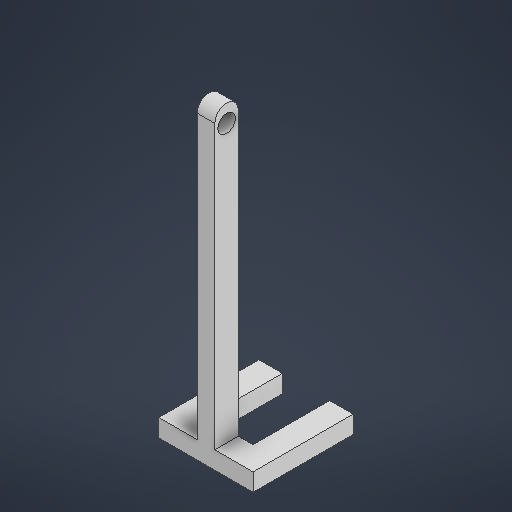
# Autodesk Inventor part: Soporte_Seguro_Tapa
Saved by Autodesk Inventor 2026 (Build 300175000, 175)
## iProperties
Created: 2025-07-02
Part Number: Soporte_Seguro_Tapa
Material: Genérico
Document SubType Name: Modeling
Designer: oscar
Density: 1 g/cm^3
Appearance: Valor por defecto
Author: oscar
Autodesk Inventor part; units mm, degrees
ref_plane "YZ Plane" through (0, 0, 0) normal (1, 0, 0) x (0, 1, 0)
ref_plane "XZ Plane" through (0, 0, 0) normal (0, 1, 0) x (-1, 0, 0)
ref_plane "XY Plane" through (0, 0, 0) normal (0, 0, 1) x (1, 0, 0)
sketch "Boceto1" plane through (0, 0, 0) normal (0, 1, 0) x (-1, 0, 0)
  line L0 (-8, 5.1855) -> (-8, -11.8145)
  line L1 (-8, -11.8145) -> (-4, -11.8145)
  line L2 (-4, -11.8145) -> (-4, 1.1855)
  line L3 (-4, 1.1855) -> (4, 1.1855)
  line L4 (4, 1.1855) -> (4, -11.8145)
  line L5 (4, -11.8145) -> (8, -11.8145)
  line L6 (8, -11.8145) -> (8, 5.1855)
  line L7 (8, 5.1855) -> (-8, 5.1855)
  point P0 (3.454, 5.1855)
  dimension "d1" = 8
  dimension "d2" = 13
  dimension "d3" = 13
  dimension "d4" = 4
  dimension "d5" = 4
  dimension "d6" = 4
  constraints: 16 end point, 6 perpendicular, 1 horizontal
  measures "d1" distance of L2.end L3.end
  measures "d2" distance of L3.end L4.end
  measures "d3" distance of L1.end L2.end
  measures "d4" distance of L4.end L5.end
  measures "d5" distance of L0.end L1.end
  measures "d6" distance from line of L3 point (3.454, 5.185)
extrude "Extrusión1" add sketch "Boceto1" along normal blind 3
sketch "Boceto2" plane through (0, 3, 0) normal (0, 1, 0) x (1, 0, 0)
  line L0 (-8, -5.1855) -> (8, -5.1855) projected
  line L1 (4, -1.1855) -> (-4, -1.1855) projected
  line L2 (-1.5, -5.1855) -> (1.5, -5.1855)
  line L3 (1.5, -5.1855) -> (1.5, -1.1855)
  line L4 (1.5, -1.1855) -> (-1.5, -1.1855)
  line L5 (-1.5, -1.1855) -> (-1.5, -5.1855)
  line L6 (-8, 11.8145) -> (-8, -5.1855) projected
  point P0 (0, 0)
  point P1 (-1.5, -3.1855)
  point P2 (0, -3.2062)
  point P3 (-1.5, -1.1855)
  dimension "d10" = 3
  dimension "d13" = 1.5
  dimension "d14" = 6.5
  constraints: 8 end point, 2 parallel, 2 point on line, 1 horizontal, 1 midpoint, 1 perpendicular
  measures "d10" distance of L4.end L3.end
  measures "d13" horizontal distance of point (-1.5, -3.185) point (0, -3.206)
  measures "d14" distance between parallel lines of L6 L5
extrude "Extrusión2" add sketch "Boceto2" along normal blind 50
fillet "Empalme1" radius 2 2 edges at (0, 53, 1.1855) (0, 53, 5.1855)
sketch "Boceto3" plane through (-1.5, 3, 1.1855) normal (-1, 0, 0) x (0, 0, 1)
  circle A0 centre (2, 47) radius 1.5
  line L0 (0, 0) -> (0, 48) projected
  arc A1 (4, 48) -> (0, 48) centre (2, 48) ccw projected
  point P0 (-1.1855, -3)
  dimension "d18" = 3
  dimension "d19" = 2
  dimension "d20" = 1
  constraints: 1 centre point
  measures "d18" diameter of A0
  measures "d19" distance from line of L0 A0.centre
  measures "d20" distance of A1.centre A0.centre
extrude "Extrusión3" cut sketch "Boceto3" against normal blind 25
sketch "Boceto5" plane through (-1.5, 3, 1.1855) normal (-1, 0, 0) x (0, 0, 1)
  line L0 (4, 0) -> (4, 48) projected
  line L1 (0, 0) -> (0, 48) projected
  line L2 (0, 41.0837) -> (0, 5.7835)
  line L3 (4, 5.7835) -> (4, 41.0837)
  spline S0 degree 2 poles (1.1837, 10.435) (1.2834, 10.5201) (1.5751, 10.6149) (1.7623, 10.6149) knots 0 0 0 1 2 2 2
  spline S1 degree 2 poles (1.7623, 10.6149) (1.9446, 10.6149) (2.24, 10.5225) (2.3397, 10.435) knots 0 0 0 1 2 2 2
  spline S2 degree 2 poles (2.3397, 10.435) (2.4442, 10.3426) (2.5439, 10.0983) (2.5439, 9.9512) knots 0 0 0 1 2 2 2
  spline S3 degree 2 poles (2.5439, 9.9512) (2.5439, 9.7992) (2.4406, 9.5561) (2.3397, 9.4674) knots 0 0 0 1 2 2 2
  spline S4 degree 2 poles (2.3397, 9.4674) (2.24, 9.3811) (1.9471, 9.2887) (1.7623, 9.2887) knots 0 0 0 1 2 2 2
  spline S5 degree 2 poles (1.7623, 9.2887) (1.5739, 9.2887) (1.287, 9.3823) (1.1837, 9.4686) knots 0 0 0 1 2 2 2
  spline S6 degree 2 poles (1.1837, 9.4686) (1.084, 9.5561) (0.9807, 9.8004) (0.9807, 9.9512) knots 0 0 0 1 2 2 2
  spline S7 degree 2 poles (0.9807, 9.9512) (0.9807, 10.1043) (1.0877, 10.3499) (1.1837, 10.435) knots 0 0 0 1 2 2 2
  spline S8 degree 2 poles (1.7623, 10.407) (1.614, 10.407) (1.3843, 10.3426) (1.3089, 10.2842) knots 0 0 0 1 2 2 2
  spline S9 degree 2 poles (1.3089, 10.2842) (1.2311, 10.2247) (1.1533, 10.0569) (1.1533, 9.9524) knots 0 0 0 1 2 2 2
  spline S10 degree 2 poles (1.1533, 9.9524) (1.1533, 9.8442) (1.2287, 9.6813) (1.3089, 9.6193) knots 0 0 0 1 2 2 2
  spline S11 degree 2 poles (1.3089, 9.6193) (1.3855, 9.5598) (1.6164, 9.4966) (1.7623, 9.4966) knots 0 0 0 1 2 2 2
  spline S12 degree 2 poles (1.7623, 9.4966) (2.0577, 9.4966) (2.3713, 9.7445) (2.3713, 9.9524) knots 0 0 0 1 2 2 2
  spline S13 degree 2 poles (2.3713, 9.9524) (2.3713, 10.1603) (2.0577, 10.407) (1.7623, 10.407) knots 0 0 0 1 2 2 2
  spline S14 degree 2 poles (2.539, 11.2518) (2.539, 11.0889) (2.471, 10.8604) (2.4223, 10.7595) knots 0 0 0 1 2 2 2
  line L4 (2.4223, 10.7595) -> (2.1719, 10.7595)
  line L5 (2.1719, 10.7595) -> (2.1719, 10.7741)
  spline S15 degree 2 poles (2.1719, 10.7741) (2.2643, 10.8726) (2.3664, 11.1218) (2.3664, 11.2372) knots 0 0 0 1 2 2 2
  spline S16 degree 2 poles (2.3664, 11.2372) (2.3664, 11.4026) (2.2291, 11.5715) (2.116, 11.5715) knots 0 0 0 1 2 2 2
  spline S17 degree 2 poles (2.116, 11.5715) (2.0261, 11.5715) (1.9142, 11.4828) (1.8863, 11.3867) knots 0 0 0 1 2 2 2
  spline S18 degree 2 poles (1.8863, 11.3867) (1.8668, 11.3175) (1.8401, 11.202) (1.8182, 11.1157) knots 0 0 0 1 2 2 2
  spline S19 degree 2 poles (1.8182, 11.1157) (1.7975, 11.0379) (1.7355, 10.9151) (1.6857, 10.8677) knots 0 0 0 1 2 2 2
  spline S20 degree 2 poles (1.6857, 10.8677) (1.6359, 10.8215) (1.5022, 10.7705) (1.4146, 10.7705) knots 0 0 0 1 2 2 2
  spline S21 degree 2 poles (1.4146, 10.7705) (1.2323, 10.7705) (0.9855, 11.0549) (0.9855, 11.2749) knots 0 0 0 1 2 2 2
  spline S22 degree 2 poles (0.9855, 11.2749) (0.9855, 11.4013) (1.0354, 11.625) (1.0828, 11.721) knots 0 0 0 1 2 2 2
  line L6 (1.0828, 11.721) -> (1.321, 11.721)
  line L7 (1.321, 11.721) -> (1.321, 11.7064)
  spline S23 degree 2 poles (1.321, 11.7064) (1.2554, 11.6347) (1.1582, 11.4111) (1.1582, 11.2883) knots 0 0 0 1 2 2 2
  spline S24 degree 2 poles (1.1582, 11.2883) (1.1582, 11.1497) (1.2882, 10.9783) (1.394, 10.9783) knots 0 0 0 1 2 2 2
  spline S25 degree 2 poles (1.394, 10.9783) (1.4888, 10.9783) (1.6018, 11.0792) (1.6274, 11.174) knots 0 0 0 1 2 2 2
  spline S26 degree 2 poles (1.6274, 11.174) (1.6444, 11.2372) (1.6881, 11.4208) (1.7064, 11.4816) knots 0 0 0 1 2 2 2
  spline S27 degree 2 poles (1.7064, 11.4816) (1.7538, 11.6359) (1.9446, 11.7794) (2.0844, 11.7794) knots 0 0 0 1 2 2 2
  spline S28 degree 2 poles (2.0844, 11.7794) (2.1731, 11.7794) (2.3433, 11.7077) (2.4029, 11.6432) knots 0 0 0 1 2 2 2
  spline S29 degree 2 poles (2.4029, 11.6432) (2.4685, 11.5715) (2.539, 11.3892) (2.539, 11.2518) knots 0 0 0 1 2 2 2
  spline S30 degree 2 poles (2.539, 12.5683) (2.539, 12.4224) (2.4406, 12.1756) (2.3421, 12.0857) knots 0 0 0 1 2 2 2
  spline S31 degree 2 poles (2.3421, 12.0857) (2.2449, 11.9957) (1.9531, 11.8973) (1.7635, 11.8973) knots 0 0 0 1 2 2 2
  spline S32 degree 2 poles (1.7635, 11.8973) (1.5751, 11.8973) (1.2955, 11.9933) (1.1922, 12.0845) knots 0 0 0 1 2 2 2
  spline S33 degree 2 poles (1.1922, 12.0845) (1.0913, 12.1744) (0.9855, 12.42) (0.9855, 12.5719) knots 0 0 0 1 2 2 2
  spline S34 degree 2 poles (0.9855, 12.5719) (0.9855, 12.6473) (1.0074, 12.7798) (1.0244, 12.8357) knots 0 0 0 1 2 2 2
  spline S35 degree 2 poles (1.0244, 12.8357) (1.0402, 12.8843) (1.0852, 12.9852) (1.112, 13.035) knots 0 0 0 1 2 2 2
  line L8 (1.112, 13.035) -> (1.3526, 13.035)
  line L9 (1.3526, 13.035) -> (1.3526, 13.0192)
  spline S36 degree 2 poles (1.3526, 13.0192) (1.3283, 12.9925) (1.2603, 12.9098) (1.2274, 12.8503) knots 0 0 0 1 2 2 2
  spline S37 degree 2 poles (1.2274, 12.8503) (1.1958, 12.7932) (1.1557, 12.6582) (1.1557, 12.5707) knots 0 0 0 1 2 2 2
  spline S38 degree 2 poles (1.1557, 12.5707) (1.1557, 12.4747) (1.2347, 12.3033) (1.3101, 12.2389) knots 0 0 0 1 2 2 2
  spline S39 degree 2 poles (1.3101, 12.2389) (1.3867, 12.1756) (1.6189, 12.1051) (1.7635, 12.1051) knots 0 0 0 1 2 2 2
  spline S40 degree 2 poles (1.7635, 12.1051) (1.9179, 12.1051) (2.1403, 12.1793) (2.2169, 12.2437) knots 0 0 0 1 2 2 2
  spline S41 degree 2 poles (2.2169, 12.2437) (2.2911, 12.3069) (2.3664, 12.4759) (2.3664, 12.5707) knots 0 0 0 1 2 2 2
  spline S42 degree 2 poles (2.3664, 12.5707) (2.3664, 12.657) (2.3239, 12.8041) (2.2923, 12.8612) knots 0 0 0 1 2 2 2
  spline S43 degree 2 poles (2.2923, 12.8612) (2.2607, 12.9159) (2.195, 12.9974) (2.1719, 13.0205) knots 0 0 0 1 2 2 2
  line L10 (2.1719, 13.0205) -> (2.1719, 13.035)
  line L11 (2.1719, 13.035) -> (2.4102, 13.035)
  spline S44 degree 2 poles (2.4102, 13.035) (2.4333, 12.9852) (2.4758, 12.8977) (2.4953, 12.8357) knots 0 0 0 1 2 2 2
  spline S45 degree 2 poles (2.4953, 12.8357) (2.5172, 12.7701) (2.539, 12.6582) (2.539, 12.5683) knots 0 0 0 1 2 2 2
  line L12 (2.5123, 13.0594) -> (1.0123, 13.565)
  line L13 (1.0123, 13.565) -> (1.0123, 13.8106)
  line L14 (1.0123, 13.8106) -> (2.5123, 14.3162)
  line L15 (2.5123, 14.3162) -> (2.5123, 14.106)
  line L16 (2.5123, 14.106) -> (2.0929, 13.9698)
  line L17 (2.0929, 13.9698) -> (2.0929, 13.3973)
  line L18 (2.0929, 13.3973) -> (2.5123, 13.2611)
  line L19 (2.5123, 13.2611) -> (2.5123, 13.0594)
  line L20 (1.9227, 13.9151) -> (1.2165, 13.6829)
  line L21 (1.2165, 13.6829) -> (1.9227, 13.452)
  line L22 (1.9227, 13.452) -> (1.9227, 13.9151)
  line L23 (2.5123, 15.6388) -> (2.5123, 15.3799)
  line L24 (2.5123, 15.3799) -> (1.9155, 14.9058)
  line L25 (1.9155, 14.9058) -> (1.9155, 14.6773)
  line L26 (1.9155, 14.6773) -> (2.5123, 14.6773)
  line L27 (2.5123, 14.6773) -> (2.5123, 14.4779)
  line L28 (2.5123, 14.4779) -> (1.0123, 14.4779)
  line L29 (1.0123, 14.4779) -> (1.0123, 14.8645)
  spline S46 degree 2 poles (1.0123, 14.8645) (1.0123, 14.9933) (1.0402, 15.1671) (1.0913, 15.2462) knots 0 0 0 1 2 2 2
  spline S47 degree 2 poles (1.0913, 15.2462) (1.1424, 15.3252) (1.3016, 15.4163) (1.4195, 15.4163) knots 0 0 0 1 2 2 2
  spline S48 degree 2 poles (1.4195, 15.4163) (1.5836, 15.4163) (1.8061, 15.2486) (1.8595, 15.1051) knots 0 0 0 1 2 2 2
  line L30 (1.8595, 15.1051) -> (2.5123, 15.6388)
  spline S49 degree 2 poles (1.4353, 15.2085) (1.3697, 15.2085) (1.2688, 15.1623) (1.236, 15.1137) knots 0 0 0 1 2 2 2
  spline S50 degree 2 poles (1.236, 15.1137) (1.208, 15.0711) (1.1849, 14.9581) (1.1849, 14.8754) knots 0 0 0 1 2 2 2
  line L31 (1.1849, 14.8754) -> (1.1849, 14.6773)
  line L32 (1.1849, 14.6773) -> (1.7489, 14.6773)
  line L33 (1.7489, 14.6773) -> (1.7489, 14.8523)
  spline S51 degree 2 poles (1.7489, 14.8523) (1.7489, 14.9386) (1.7185, 15.076) (1.6711, 15.1234) knots 0 0 0 1 2 2 2
  spline S52 degree 2 poles (1.6711, 15.1234) (1.6298, 15.1671) (1.5131, 15.2085) (1.4353, 15.2085) knots 0 0 0 1 2 2 2
  line L34 (2.9073, 16.7279) -> (2.9073, 16.5602)
  line L35 (2.9073, 16.5602) -> (0.9454, 16.5602)
  line L36 (0.9454, 16.5602) -> (0.9454, 16.7279)
  line L37 (0.9454, 16.7279) -> (2.9073, 16.7279)
  line L38 (2.5123, 18.358) -> (2.5123, 17.7769)
  line L39 (2.5123, 17.7769) -> (2.3591, 17.7769)
  line L40 (2.3591, 17.7769) -> (2.3591, 17.9678)
  line L41 (2.3591, 17.9678) -> (1.1655, 17.9678)
  line L42 (1.1655, 17.9678) -> (1.1655, 17.7769)
  line L43 (1.1655, 17.7769) -> (1.0123, 17.7769)
  line L44 (1.0123, 17.7769) -> (1.0123, 18.358)
  line L45 (1.0123, 18.358) -> (1.1655, 18.358)
  line L46 (1.1655, 18.358) -> (1.1655, 18.1671)
  line L47 (1.1655, 18.1671) -> (2.3591, 18.1671)
  line L48 (2.3591, 18.1671) -> (2.3591, 18.358)
  line L49 (2.3591, 18.358) -> (2.5123, 18.358)
  line L50 (2.5123, 19.7656) -> (2.5123, 19.5067)
  line L51 (2.5123, 19.5067) -> (1.9155, 19.0326)
  line L52 (1.9155, 19.0326) -> (1.9155, 18.8041)
  line L53 (1.9155, 18.8041) -> (2.5123, 18.8041)
  line L54 (2.5123, 18.8041) -> (2.5123, 18.6047)
  line L55 (2.5123, 18.6047) -> (1.0123, 18.6047)
  line L56 (1.0123, 18.6047) -> (1.0123, 18.9913)
  spline S53 degree 2 poles (1.0123, 18.9913) (1.0123, 19.1201) (1.0402, 19.294) (1.0913, 19.373) knots 0 0 0 1 2 2 2
  spline S54 degree 2 poles (1.0913, 19.373) (1.1424, 19.452) (1.3016, 19.5432) (1.4195, 19.5432) knots 0 0 0 1 2 2 2
  spline S55 degree 2 poles (1.4195, 19.5432) (1.5836, 19.5432) (1.8061, 19.3754) (1.8595, 19.232) knots 0 0 0 1 2 2 2
  line L57 (1.8595, 19.232) -> (2.5123, 19.7656)
  spline S56 degree 2 poles (1.4353, 19.3353) (1.3697, 19.3353) (1.2688, 19.2891) (1.236, 19.2405) knots 0 0 0 1 2 2 2
  spline S57 degree 2 poles (1.236, 19.2405) (1.208, 19.1979) (1.1849, 19.0849) (1.1849, 19.0022) knots 0 0 0 1 2 2 2
  line L58 (1.1849, 19.0022) -> (1.1849, 18.8041)
  line L59 (1.1849, 18.8041) -> (1.7489, 18.8041)
  line L60 (1.7489, 18.8041) -> (1.7489, 18.9791)
  spline S58 degree 2 poles (1.7489, 18.9791) (1.7489, 19.0654) (1.7185, 19.2028) (1.6711, 19.2502) knots 0 0 0 1 2 2 2
  spline S59 degree 2 poles (1.6711, 19.2502) (1.6298, 19.294) (1.5131, 19.3353) (1.4353, 19.3353) knots 0 0 0 1 2 2 2
  line L61 (2.5123, 21.1708) -> (2.5123, 20.9714)
  line L62 (2.5123, 20.9714) -> (1.2202, 20.9714)
  line L63 (1.2202, 20.9714) -> (2.099, 20.58)
  line L64 (2.099, 20.58) -> (2.099, 20.4585)
  line L65 (2.099, 20.4585) -> (1.2202, 20.0707)
  line L66 (1.2202, 20.0707) -> (2.5123, 20.0707)
  line L67 (2.5123, 20.0707) -> (2.5123, 19.8847)
  line L68 (2.5123, 19.8847) -> (1.0123, 19.8847)
  line L69 (1.0123, 19.8847) -> (1.0123, 20.157)
  line L70 (1.0123, 20.157) -> (1.8474, 20.5314)
  line L71 (1.8474, 20.5314) -> (1.0123, 20.8936)
  line L72 (1.0123, 20.8936) -> (1.0123, 21.1708)
  line L73 (1.0123, 21.1708) -> (2.5123, 21.1708)
  line L74 (2.5123, 21.313) -> (1.0123, 21.8187)
  line L75 (1.0123, 21.8187) -> (1.0123, 22.0642)
  line L76 (1.0123, 22.0642) -> (2.5123, 22.5699)
  line L77 (2.5123, 22.5699) -> (2.5123, 22.3596)
  line L78 (2.5123, 22.3596) -> (2.0929, 22.2235)
  line L79 (2.0929, 22.2235) -> (2.0929, 21.6509)
  line L80 (2.0929, 21.6509) -> (2.5123, 21.5148)
  line L81 (2.5123, 21.5148) -> (2.5123, 21.313)
  line L82 (1.9227, 22.1688) -> (1.2165, 21.9366)
  line L83 (1.2165, 21.9366) -> (1.9227, 21.7056)
  line L84 (1.9227, 21.7056) -> (1.9227, 22.1688)
  line L85 (2.9073, 23.7016) -> (2.9073, 23.5338)
  line L86 (2.9073, 23.5338) -> (0.9454, 23.5338)
  line L87 (0.9454, 23.5338) -> (0.9454, 23.7016)
  line L88 (0.9454, 23.7016) -> (2.9073, 23.7016)
  spline S60 degree 2 poles (2.539, 25.3949) (2.539, 25.249) (2.4406, 25.0022) (2.3421, 24.9123) knots 0 0 0 1 2 2 2
  spline S61 degree 2 poles (2.3421, 24.9123) (2.2449, 24.8223) (1.9531, 24.7239) (1.7635, 24.7239) knots 0 0 0 1 2 2 2
  spline S62 degree 2 poles (1.7635, 24.7239) (1.5751, 24.7239) (1.2955, 24.8199) (1.1922, 24.9111) knots 0 0 0 1 2 2 2
  spline S63 degree 2 poles (1.1922, 24.9111) (1.0913, 25.001) (0.9855, 25.2466) (0.9855, 25.3985) knots 0 0 0 1 2 2 2
  spline S64 degree 2 poles (0.9855, 25.3985) (0.9855, 25.4739) (1.0074, 25.6064) (1.0244, 25.6623) knots 0 0 0 1 2 2 2
  spline S65 degree 2 poles (1.0244, 25.6623) (1.0402, 25.7109) (1.0852, 25.8118) (1.112, 25.8616) knots 0 0 0 1 2 2 2
  line L89 (1.112, 25.8616) -> (1.3526, 25.8616)
  line L90 (1.3526, 25.8616) -> (1.3526, 25.8458)
  spline S66 degree 2 poles (1.3526, 25.8458) (1.3283, 25.8191) (1.2603, 25.7364) (1.2274, 25.6769) knots 0 0 0 1 2 2 2
  spline S67 degree 2 poles (1.2274, 25.6769) (1.1958, 25.6197) (1.1557, 25.4848) (1.1557, 25.3973) knots 0 0 0 1 2 2 2
  spline S68 degree 2 poles (1.1557, 25.3973) (1.1557, 25.3013) (1.2347, 25.1299) (1.3101, 25.0654) knots 0 0 0 1 2 2 2
  spline S69 degree 2 poles (1.3101, 25.0654) (1.3867, 25.0022) (1.6189, 24.9317) (1.7635, 24.9317) knots 0 0 0 1 2 2 2
  spline S70 degree 2 poles (1.7635, 24.9317) (1.9179, 24.9317) (2.1403, 25.0059) (2.2169, 25.0703) knots 0 0 0 1 2 2 2
  spline S71 degree 2 poles (2.2169, 25.0703) (2.2911, 25.1335) (2.3664, 25.3025) (2.3664, 25.3973) knots 0 0 0 1 2 2 2
  spline S72 degree 2 poles (2.3664, 25.3973) (2.3664, 25.4836) (2.3239, 25.6307) (2.2923, 25.6878) knots 0 0 0 1 2 2 2
  spline S73 degree 2 poles (2.2923, 25.6878) (2.2607, 25.7425) (2.195, 25.8239) (2.1719, 25.847) knots 0 0 0 1 2 2 2
  line L91 (2.1719, 25.847) -> (2.1719, 25.8616)
  line L92 (2.1719, 25.8616) -> (2.4102, 25.8616)
  spline S74 degree 2 poles (2.4102, 25.8616) (2.4333, 25.8118) (2.4758, 25.7243) (2.4953, 25.6623) knots 0 0 0 1 2 2 2
  spline S75 degree 2 poles (2.4953, 25.6623) (2.5172, 25.5966) (2.539, 25.4848) (2.539, 25.3949) knots 0 0 0 1 2 2 2
  line L93 (2.5123, 27.1368) -> (2.5123, 26.9374)
  line L94 (2.5123, 26.9374) -> (1.7781, 26.9374)
  line L95 (1.7781, 26.9374) -> (1.7781, 26.247)
  line L96 (1.7781, 26.247) -> (2.5123, 26.247)
  line L97 (2.5123, 26.247) -> (2.5123, 26.0476)
  line L98 (2.5123, 26.0476) -> (1.0123, 26.0476)
  line L99 (1.0123, 26.0476) -> (1.0123, 26.247)
  line L100 (1.0123, 26.247) -> (1.6006, 26.247)
  line L101 (1.6006, 26.247) -> (1.6006, 26.9374)
  line L102 (1.6006, 26.9374) -> (1.0123, 26.9374)
  line L103 (1.0123, 26.9374) -> (1.0123, 27.1368)
  line L104 (1.0123, 27.1368) -> (2.5123, 27.1368)
  line L105 (2.5123, 27.4406) -> (1.0123, 27.4406)
  line L106 (1.0123, 27.4406) -> (1.0123, 28.3791)
  line L107 (1.0123, 28.3791) -> (1.1898, 28.3791)
  line L108 (1.1898, 28.3791) -> (1.1898, 27.64)
  line L109 (1.1898, 27.64) -> (1.6006, 27.64)
  line L110 (1.6006, 27.64) -> (1.6006, 28.3292)
  line L111 (1.6006, 28.3292) -> (1.7781, 28.3292)
  line L112 (1.7781, 28.3292) -> (1.7781, 27.64)
  line L113 (1.7781, 27.64) -> (2.3348, 27.64)
  line L114 (2.3348, 27.64) -> (2.3348, 28.3791)
  line L115 (2.3348, 28.3791) -> (2.5123, 28.3791)
  line L116 (2.5123, 28.3791) -> (2.5123, 27.4406)
  spline S76 degree 2 poles (2.539, 29.1838) (2.539, 29.0379) (2.4406, 28.7911) (2.3421, 28.7012) knots 0 0 0 1 2 2 2
  spline S77 degree 2 poles (2.3421, 28.7012) (2.2449, 28.6112) (1.9531, 28.5128) (1.7635, 28.5128) knots 0 0 0 1 2 2 2
  spline S78 degree 2 poles (1.7635, 28.5128) (1.5751, 28.5128) (1.2955, 28.6088) (1.1922, 28.7) knots 0 0 0 1 2 2 2
  spline S79 degree 2 poles (1.1922, 28.7) (1.0913, 28.7899) (0.9855, 29.0355) (0.9855, 29.1874) knots 0 0 0 1 2 2 2
  spline S80 degree 2 poles (0.9855, 29.1874) (0.9855, 29.2628) (1.0074, 29.3953) (1.0244, 29.4512) knots 0 0 0 1 2 2 2
  spline S81 degree 2 poles (1.0244, 29.4512) (1.0402, 29.4998) (1.0852, 29.6007) (1.112, 29.6505) knots 0 0 0 1 2 2 2
  line L117 (1.112, 29.6505) -> (1.3526, 29.6505)
  line L118 (1.3526, 29.6505) -> (1.3526, 29.6347)
  spline S82 degree 2 poles (1.3526, 29.6347) (1.3283, 29.608) (1.2603, 29.5253) (1.2274, 29.4658) knots 0 0 0 1 2 2 2
  spline S83 degree 2 poles (1.2274, 29.4658) (1.1958, 29.4086) (1.1557, 29.2737) (1.1557, 29.1862) knots 0 0 0 1 2 2 2
  spline S84 degree 2 poles (1.1557, 29.1862) (1.1557, 29.0902) (1.2347, 28.9188) (1.3101, 28.8543) knots 0 0 0 1 2 2 2
  spline S85 degree 2 poles (1.3101, 28.8543) (1.3867, 28.7911) (1.6189, 28.7206) (1.7635, 28.7206) knots 0 0 0 1 2 2 2
  spline S86 degree 2 poles (1.7635, 28.7206) (1.9179, 28.7206) (2.1403, 28.7948) (2.2169, 28.8592) knots 0 0 0 1 2 2 2
  spline S87 degree 2 poles (2.2169, 28.8592) (2.2911, 28.9224) (2.3664, 29.0914) (2.3664, 29.1862) knots 0 0 0 1 2 2 2
  spline S88 degree 2 poles (2.3664, 29.1862) (2.3664, 29.2725) (2.3239, 29.4196) (2.2923, 29.4767) knots 0 0 0 1 2 2 2
  spline S89 degree 2 poles (2.2923, 29.4767) (2.2607, 29.5314) (2.195, 29.6128) (2.1719, 29.6359) knots 0 0 0 1 2 2 2
  line L119 (2.1719, 29.6359) -> (2.1719, 29.6505)
  line L120 (2.1719, 29.6505) -> (2.4102, 29.6505)
  spline S90 degree 2 poles (2.4102, 29.6505) (2.4333, 29.6007) (2.4758, 29.5132) (2.4953, 29.4512) knots 0 0 0 1 2 2 2
  spline S91 degree 2 poles (2.4953, 29.4512) (2.5172, 29.3855) (2.539, 29.2737) (2.539, 29.1838) knots 0 0 0 1 2 2 2
  line L121 (2.5123, 30.9256) -> (2.5123, 30.7263)
  line L122 (2.5123, 30.7263) -> (1.7781, 30.7263)
  line L123 (1.7781, 30.7263) -> (1.7781, 30.0359)
  line L124 (1.7781, 30.0359) -> (2.5123, 30.0359)
  line L125 (2.5123, 30.0359) -> (2.5123, 29.8365)
  line L126 (2.5123, 29.8365) -> (1.0123, 29.8365)
  line L127 (1.0123, 29.8365) -> (1.0123, 30.0359)
  line L128 (1.0123, 30.0359) -> (1.6006, 30.0359)
  line L129 (1.6006, 30.0359) -> (1.6006, 30.7263)
  line L130 (1.6006, 30.7263) -> (1.0123, 30.7263)
  line L131 (1.0123, 30.7263) -> (1.0123, 30.9256)
  line L132 (1.0123, 30.9256) -> (2.5123, 30.9256)
  spline S92 degree 2 poles (1.1837, 32.2907) (1.2834, 32.3758) (1.5751, 32.4706) (1.7623, 32.4706) knots 0 0 0 1 2 2 2
  spline S93 degree 2 poles (1.7623, 32.4706) (1.9446, 32.4706) (2.24, 32.3782) (2.3397, 32.2907) knots 0 0 0 1 2 2 2
  spline S94 degree 2 poles (2.3397, 32.2907) (2.4442, 32.1983) (2.5439, 31.954) (2.5439, 31.8069) knots 0 0 0 1 2 2 2
  spline S95 degree 2 poles (2.5439, 31.8069) (2.5439, 31.655) (2.4406, 31.4119) (2.3397, 31.3231) knots 0 0 0 1 2 2 2
  spline S96 degree 2 poles (2.3397, 31.3231) (2.24, 31.2368) (1.9471, 31.1444) (1.7623, 31.1444) knots 0 0 0 1 2 2 2
  spline S97 degree 2 poles (1.7623, 31.1444) (1.5739, 31.1444) (1.287, 31.238) (1.1837, 31.3244) knots 0 0 0 1 2 2 2
  spline S98 degree 2 poles (1.1837, 31.3244) (1.084, 31.4119) (0.9807, 31.6562) (0.9807, 31.8069) knots 0 0 0 1 2 2 2
  spline S99 degree 2 poles (0.9807, 31.8069) (0.9807, 31.9601) (1.0877, 32.2056) (1.1837, 32.2907) knots 0 0 0 1 2 2 2
  spline S100 degree 2 poles (1.7623, 32.2628) (1.614, 32.2628) (1.3843, 32.1983) (1.3089, 32.14) knots 0 0 0 1 2 2 2
  spline S101 degree 2 poles (1.3089, 32.14) (1.2311, 32.0804) (1.1533, 31.9127) (1.1533, 31.8081) knots 0 0 0 1 2 2 2
  spline S102 degree 2 poles (1.1533, 31.8081) (1.1533, 31.7) (1.2287, 31.5371) (1.3089, 31.4751) knots 0 0 0 1 2 2 2
  spline S103 degree 2 poles (1.3089, 31.4751) (1.3855, 31.4155) (1.6164, 31.3523) (1.7623, 31.3523) knots 0 0 0 1 2 2 2
  spline S104 degree 2 poles (1.7623, 31.3523) (2.0577, 31.3523) (2.3713, 31.6003) (2.3713, 31.8081) knots 0 0 0 1 2 2 2
  spline S105 degree 2 poles (2.3713, 31.8081) (2.3713, 32.016) (2.0577, 32.2628) (1.7623, 32.2628) knots 0 0 0 1 2 2 2
  line L133 (2.9073, 33.6594) -> (2.9073, 33.4917)
  line L134 (2.9073, 33.4917) -> (0.9454, 33.4917)
  line L135 (0.9454, 33.4917) -> (0.9454, 33.6594)
  line L136 (0.9454, 33.6594) -> (2.9073, 33.6594)
  spline S106 degree 2 poles (1.4645, 35.715) (1.5617, 35.715) (1.7368, 35.6457) (1.7975, 35.5837) knots 0 0 0 1 2 2 2
  spline S107 degree 2 poles (1.7975, 35.5837) (1.8741, 35.5059) (1.9531, 35.2956) (1.9531, 35.1351) knots 0 0 0 1 2 2 2
  line L137 (1.9531, 35.1351) -> (1.9531, 34.9662)
  line L138 (1.9531, 34.9662) -> (2.5123, 34.9662)
  line L139 (2.5123, 34.9662) -> (2.5123, 34.7668)
  line L140 (2.5123, 34.7668) -> (1.0123, 34.7668)
  line L141 (1.0123, 34.7668) -> (1.0123, 35.1436)
  spline S108 degree 2 poles (1.0123, 35.1436) (1.0123, 35.2774) (1.0561, 35.4645) (1.1059, 35.5363) knots 0 0 0 1 2 2 2
  spline S109 degree 2 poles (1.1059, 35.5363) (1.163, 35.6201) (1.3393, 35.715) (1.4645, 35.715) knots 0 0 0 1 2 2 2
  spline S110 degree 2 poles (1.4706, 35.5071) (1.3928, 35.5071) (1.2785, 35.4536) (1.242, 35.3989) knots 0 0 0 1 2 2 2
  spline S111 degree 2 poles (1.242, 35.3989) (1.2104, 35.3515) (1.1849, 35.2251) (1.1849, 35.1315) knots 0 0 0 1 2 2 2
  line L142 (1.1849, 35.1315) -> (1.1849, 34.9662)
  line L143 (1.1849, 34.9662) -> (1.783, 34.9662)
  line L144 (1.783, 34.9662) -> (1.783, 35.1023)
  spline S112 degree 2 poles (1.783, 35.1023) (1.783, 35.2239) (1.7441, 35.3734) (1.693, 35.422) knots 0 0 0 1 2 2 2
  spline S113 degree 2 poles (1.693, 35.422) (1.648, 35.467) (1.5423, 35.5071) (1.4706, 35.5071) knots 0 0 0 1 2 2 2
  line L145 (2.5123, 36.4273) -> (2.5123, 35.8462)
  line L146 (2.5123, 35.8462) -> (2.3591, 35.8462)
  line L147 (2.3591, 35.8462) -> (2.3591, 36.0371)
  line L148 (2.3591, 36.0371) -> (1.1655, 36.0371)
  line L149 (1.1655, 36.0371) -> (1.1655, 35.8462)
  line L150 (1.1655, 35.8462) -> (1.0123, 35.8462)
  line L151 (1.0123, 35.8462) -> (1.0123, 36.4273)
  line L152 (1.0123, 36.4273) -> (1.1655, 36.4273)
  line L153 (1.1655, 36.4273) -> (1.1655, 36.2364)
  line L154 (1.1655, 36.2364) -> (2.3591, 36.2364)
  line L155 (2.3591, 36.2364) -> (2.3591, 36.4273)
  line L156 (2.3591, 36.4273) -> (2.5123, 36.4273)
  spline S114 degree 2 poles (1.4645, 37.6222) (1.5617, 37.6222) (1.7368, 37.5529) (1.7975, 37.4909) knots 0 0 0 1 2 2 2
  spline S115 degree 2 poles (1.7975, 37.4909) (1.8741, 37.4131) (1.9531, 37.2028) (1.9531, 37.0423) knots 0 0 0 1 2 2 2
  line L157 (1.9531, 37.0423) -> (1.9531, 36.8734)
  line L158 (1.9531, 36.8734) -> (2.5123, 36.8734)
  line L159 (2.5123, 36.8734) -> (2.5123, 36.674)
  line L160 (2.5123, 36.674) -> (1.0123, 36.674)
  line L161 (1.0123, 36.674) -> (1.0123, 37.0509)
  spline S116 degree 2 poles (1.0123, 37.0509) (1.0123, 37.1846) (1.0561, 37.3718) (1.1059, 37.4435) knots 0 0 0 1 2 2 2
  spline S117 degree 2 poles (1.1059, 37.4435) (1.163, 37.5274) (1.3393, 37.6222) (1.4645, 37.6222) knots 0 0 0 1 2 2 2
  spline S118 degree 2 poles (1.4706, 37.4143) (1.3928, 37.4143) (1.2785, 37.3608) (1.242, 37.3061) knots 0 0 0 1 2 2 2
  spline S119 degree 2 poles (1.242, 37.3061) (1.2104, 37.2587) (1.1849, 37.1323) (1.1849, 37.0387) knots 0 0 0 1 2 2 2
  line L162 (1.1849, 37.0387) -> (1.1849, 36.8734)
  line L163 (1.1849, 36.8734) -> (1.783, 36.8734)
  line L164 (1.783, 36.8734) -> (1.783, 37.0095)
  spline S120 degree 2 poles (1.783, 37.0095) (1.783, 37.1311) (1.7441, 37.2806) (1.693, 37.3292) knots 0 0 0 1 2 2 2
  spline S121 degree 2 poles (1.693, 37.3292) (1.648, 37.3742) (1.5423, 37.4143) (1.4706, 37.4143) knots 0 0 0 1 2 2 2
  line L165 (2.5123, 37.8118) -> (1.0123, 37.8118)
  line L166 (1.0123, 37.8118) -> (1.0123, 38.7502)
  line L167 (1.0123, 38.7502) -> (1.1898, 38.7502)
  line L168 (1.1898, 38.7502) -> (1.1898, 38.0111)
  line L169 (1.1898, 38.0111) -> (1.6006, 38.0111)
  line L170 (1.6006, 38.0111) -> (1.6006, 38.7004)
  line L171 (1.6006, 38.7004) -> (1.7781, 38.7004)
  line L172 (1.7781, 38.7004) -> (1.7781, 38.0111)
  line L173 (1.7781, 38.0111) -> (2.3348, 38.0111)
  line L174 (2.3348, 38.0111) -> (2.3348, 38.7502)
  line L175 (2.3348, 38.7502) -> (2.5123, 38.7502)
  line L176 (2.5123, 38.7502) -> (2.5123, 37.8118)
  point P0 (-1.1855, -3)
  dimension "d1" = 8
  dimension "d2" = 13
  dimension "d3" = 13
  dimension "d4" = 4
  dimension "d5" = 4
  dimension "d6" = 4
  constraints: 4 end point, 2 point on line, 1 parallel, 1 vertical
extrude "Extrusión5" cut sketch "Boceto5" against normal blind 1
equation "\"d3\" = d2"
equation "\"d5\" = d4"
